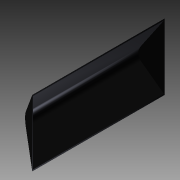
# Autodesk Inventor part: front bumper
Saved by Autodesk Inventor 2012 (Build 160160000, 160)
## iProperties
Created: 2011-12-02
Part Number: front bumper
Material: Default
Document SubType Name: Modeling
Designer: Antonella
Density: 1 g/cm^3
Author: Antonella
Autodesk Inventor part; units mm, degrees
ref_plane "YZ Plane" through (0, 0, 0) normal (1, 0, 0) x (0, 1, 0)
ref_plane "XZ Plane" through (0, 0, 0) normal (0, 1, 0) x (-1, 0, 0)
ref_plane "XY Plane" through (0, 0, 0) normal (0, 0, 1) x (1, 0, 0)
sketch "Sketch1" plane through (0, 0, 0) normal (0, 0, 1) x (1, 0, 0)
  line L0 (-93.9216, 0) -> (15.6536, 0) projected
  line L1 (0, -306.9874) -> (0, 252.5784) projected
  line L2 (0, 152.4) -> (0, -152.4)
  line L3 (0, 152.4) -> (-69.85, 31.4163)
  line L4 (0, -152.4) -> (-69.85, -31.4163)
  arc A0 (-69.85, 31.4163) -> (-69.85, -31.4163) centre (-15.4355, 0) ccw
  line L5 (-78.268, 172.6404) -> (-78.268, -227.0494) construction
  point P0 (0, 0)
  point P1 (0, 0)
  dimension "d0" = 304.8
  dimension "d13" = 30
  dimension "d14" = 139.7
  constraints: 8 end point, 3 tangent, 2 point on circle, 2 point on line, 1 centre point, 1 coincident, 1 equal length, 1 midpoint, 1 parallel
  measures "d0" distance of L2.start L2.end
  measures "d13" angle of L1 L3
  measures "d14" distance of L2.start L3.end
extrude "Extrusion1" add sketch "Sketch1" along normal mid plane 609.6
sketch "Sketch3" plane through (0, 0, 0) normal (0, 1, 0) x (-1, 0, 0)
  line L0 (69.85, 304.8) -> (0, 304.8) projected
  line L1 (0, -304.8) -> (0, 304.8) projected
  line L2 (69.85, 304.8) -> (69.85, 304.8) projected
  line L3 (69.85, -304.8) -> (69.85, 304.8) projected
  line L4 (69.85, -304.8) -> (69.85, -304.8) projected
  line L5 (69.85, -304.8) -> (69.85, 304.8) projected
  line L6 (78.268, -304.8) -> (78.268, 304.8) projected
  line L7 (69.85, 304.8) -> (78.268, 304.8) projected
  line L8 (0, 304.8) -> (78.268, 259.612)
  point P0 (0, 0)
  dimension "d8" = 30
  constraints: 2 end point, 1 point on line
  measures "d8" angle of L0 L8
extrude "Extrusion3" cut sketch "Sketch3" along normal through all both and the other way through all
mirror "Mirror1" about plane through (0, 0, 0) normal (0, 0, 1) of "Extrusion3"
shell "Shell1" thickness 3.175 removed faces 1 at (0, -50.8, -101.6)
body "Solid1"
